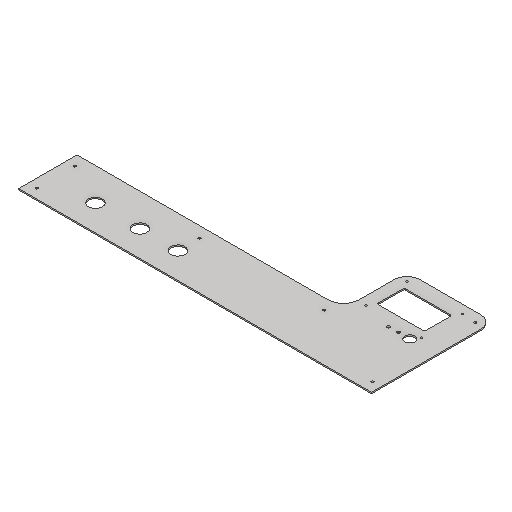
# Autodesk Inventor part: LC_ALU_2mm_Front_Plate
Saved by Autodesk Inventor 2026.1 (Build 301233000, 233)
## iProperties
Created: 2016-06-25
Part Number: LC_ALU_2mm_Front_Plate
Material: Ogólny
Document SubType Name: Modeling
Designer: Andrzej
Density: 1 g/cm^3
Appearance: Obrobione - aluminium
Mass: 122.829 g
Surface Area: 1265.9 cm^2
Volume: 122.829 cm^3
Author: Andrzej
Autodesk Inventor part; units mm, degrees
ref_plane "YZ Plane" through (0, 0, 0) normal (1, 0, 0) x (0, 1, 0)
ref_plane "XZ Plane" through (0, 0, 0) normal (0, 1, 0) x (-1, 0, 0)
ref_plane "XY Plane" through (0, 0, 0) normal (0, 0, 1) x (1, 0, 0)
sketch "Szkic1" plane through (0, 0, 0) normal (0, 0, 1) x (1, 0, 0)
  line L0 (-20.451, -12.8135) -> (535.549, -12.8135)
  line L1 (535.549, -12.8135) -> (535.549, 159.1865)
  line L2 (515.549, 179.1865) -> (419.549, 179.1865)
  line L3 (399.549, 159.1865) -> (399.549, 104.1865)
  line L4 (374.549, 79.1865) -> (-20.451, 79.1865)
  line L5 (-20.451, 79.1865) -> (-20.451, -12.8135)
  line L6 (419.049, 155.1865) -> (494.049, 155.1865)
  line L7 (494.049, 155.1865) -> (494.049, 112.1865)
  line L8 (494.049, 112.1865) -> (419.049, 112.1865)
  line L9 (419.049, 112.1865) -> (419.049, 155.1865)
  arc A0 (374.549, 79.1865) -> (399.549, 104.1865) centre (374.549, 104.1865) ccw
  arc A1 (419.549, 179.1865) -> (399.549, 159.1865) centre (419.549, 159.1865) ccw
  arc A2 (535.549, 159.1865) -> (515.549, 179.1865) centre (515.549, 159.1865) ccw
  circle A3 centre (493.049, 90.1865) radius 8
  circle A4 centre (475.049, 90.1865) radius 2.5
  circle A5 centre (459.849, 90.1865) radius 2.5
  circle A6 centre (189.549, 28.1865) radius 11
  circle A7 centre (129.549, 28.1865) radius 11
  circle A8 centre (59.549, 28.1865) radius 11
  point P0 (0, 0)
  point P1 (535.549, 179.1865)
  point P2 (399.549, 179.1865)
  point P3 (399.549, 79.1865)
  point P4 (500.549, 166.1865)
  point P5 (500.549, 101.1865)
  point P6 (412.549, 101.1865)
  point P7 (412.549, 166.1865)
  point P8 (386.049, 62.1865)
  point P9 (522.049, 164.1865)
  point P10 (522.049, 2.1865)
  point P11 (-6.951, 2.1865)
  point P12 (-6.951, 62.1865)
  point P13 (189.549, 62.1865)
  dimension "d0" = 556
  dimension "d1" = 92
  dimension "d2" = 100
  dimension "d3" = 136
  dimension "d6" = 75
  dimension "d7" = 43
  dimension "d8" = 24
  dimension "d12" = 25
  dimension "d13" = 20
  dimension "d14" = 20
  dimension "d15" = 41.5
  dimension "d18" = 6.5
  dimension "d19" = 6.5
  dimension "d20" = 6.5
  dimension "d21" = 6.5
  dimension "d22" = 11
  dimension "d23" = 11
  dimension "d24" = 11
  dimension "d25" = 11
  dimension "d33" = 16
  dimension "d34" = 5
  dimension "d35" = 5
  dimension "d40" = 18
  dimension "d41" = 15.2
  dimension "d44" = 13.5
  dimension "d45" = 13.5
  dimension "d46" = 13.5
  dimension "d47" = 13.5
  dimension "d48" = 17
  dimension "d49" = 17
  dimension "d50" = 17
  dimension "d58" = 15
  dimension "d59" = 15
  dimension "d60" = 15
  dimension "d61" = 13.5
  dimension "d62" = 393
  dimension "d63" = 196.5
  dimension "d64" = 22
  dimension "d65" = 22
  dimension "d66" = 22
  dimension "d67" = 41
  dimension "d68" = 41
  dimension "d69" = 41
  dimension "d71" = 70
  dimension "d72" = 60
  dimension "d73" = 80
  dimension "d74" = 88
  dimension "d75" = 65
  dimension "d79" = 65
  dimension "d80" = 7.5
  dimension "d81" = 11
  dimension "d82" = 11
  dimension "d83" = 11
  constraints: 22 end point, 9 centre point, 6 perpendicular, 6 point on circle, 6 point on line, 6 tangent, 2 horizontal, 2 parallel
  measures "d0" distance of L0.start L0.end
  measures "d1" distance of L4.end L0.start
  measures "d2" distance of point (399.549, 179.187) point (399.549, 79.187)
  measures "d3" distance of point (535.549, 179.187) point (399.549, 179.187)
  measures "d6" distance of L6.start L6.end
  measures "d7" distance of L8.end L6.start
  measures "d8" distance between parallel lines of L2 L6
  measures "d12" radius of A0
  measures "d13" radius of A1
  measures "d14" radius of A2
  measures "d15" distance between parallel lines of L1 L7
  measures "d18" distance from line of L9 point (412.549, 166.187)
  measures "d19" distance from line of L9 point (412.549, 101.187)
  measures "d20" distance from line of point (500.549, 101.187) L7
  measures "d21" distance from line of L7 point (500.549, 166.187)
  measures "d22" distance from line of L6 point (412.549, 166.187)
  measures "d23" distance from line of L8 point (412.549, 101.187)
  measures "d24" distance from line of L8 point (500.549, 101.187)
  measures "d25" distance from line of L6 point (500.549, 166.187)
  measures "d33" diameter of A3
  measures "d34" diameter of A4
  measures "d35" diameter of A5
  measures "d40" distance of A4.centre A3.centre
  measures "d41" distance of A5.centre A4.centre
  measures "d44" distance from line of L1 point (522.049, 2.187)
  measures "d45" distance from line of L1 point (522.049, 164.187)
  measures "d46" distance from line of L5 point (-6.951, 62.187)
  measures "d47" distance from line of L5 point (-6.951, 2.187)
  measures "d48" distance from line of L4 point (189.549, 62.187)
  measures "d49" distance from line of L4 point (-6.951, 62.187)
  measures "d50" distance from line of point (386.049, 62.187) L4
  measures "d58" distance from line of L0 point (522.049, 2.187)
  measures "d59" distance from line of L0 point (-6.951, 2.187)
  measures "d60" distance from line of L2 point (522.049, 164.187)
  measures "d61" distance from line of point (386.049, 62.187) L3
  measures "d62" distance of point (-6.951, 62.187) point (386.049, 62.187)
  measures "d63" distance of point (189.549, 62.187) point (386.049, 62.187)
  measures "d64" diameter of A6
  measures "d65" diameter of A7
  measures "d66" diameter of A8
  measures "d67" distance from line of L0 A6.centre
  measures "d68" distance from line of L0 A7.centre
  measures "d69" distance from line of L0 A8.centre
  measures "d71" distance of A7.centre A8.centre
  measures "d72" distance of A6.centre A7.centre
  measures "d73" distance from line of L5 A8.centre
  measures "d74" distance of point (500.549, 166.187) point (412.549, 166.187)
  measures "d75" distance of point (412.549, 166.187) point (412.549, 101.187)
  measures "d79" distance of point (500.549, 166.187) point (500.549, 101.187)
  measures "d80" horizontal distance of point (500.549, 101.187) A3.centre
  measures "d81" vertical distance of point (500.549, 101.187) A3.centre
  measures "d82" vertical distance of point (500.549, 101.187) A4.centre
  measures "d83" vertical distance of point (500.549, 101.187) A5.centre
extrude "Wyciągnięcie proste2" add sketch "Szkic1" along normal blind 2 contours L5 L4 A0 L3 A1 L2 A2 L1 L0 | A3 | A4 | A5 | A6 | A7 | A8
fillet "Zaokrąglenie1" radius 2 4 edges at (419.049, 112.1865, 1) (494.049, 112.1865, 1) (494.049, 155.1865, 1) (419.049, 155.1865, 1)
hole "Otwór1" at (500.549, 166.1865, 0) at (500.549, 101.1865, 0) at (412.549, 101.1865, 0) at (412.549, 166.1865, 0) direction (0, 0, 1) diameter 3 end through all
extrude "Wyciągnięcie proste3" cut sketch "Szkic1" along normal blind 10 contours A3 | A4 | A5 | A6 | A7 | A8
hole "Otwór2" at (386.049, 62.1865, 0) at (522.049, 164.1865, 0) at (522.049, 2.1865, 0) at (-6.951, 2.1865, 0) at (-6.951, 62.1865, 0) at (189.549, 62.1865, 0) direction (0, 0, 1) diameter 4 end through all
equation "\"d23\" = d22"
equation "\"d24\" = d22"
equation "\"d25\" = d22"
equation "\"d45\" = d44"
equation "\"d46\" = d44"
equation "\"d47\" = d44"
equation "\"d50\" = d48"
equation "\"d59\" = d58"
equation "\"d61\" = d46"
equation "\"d63\" = 0.5 * d62"
equation "\"d68\" = d67"
equation "\"d69\" = d67"
